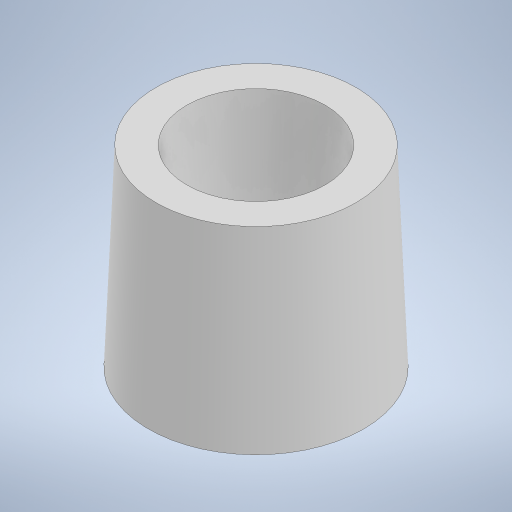
# Autodesk Inventor part: Washing Machine Base and Lid
Saved by Autodesk Inventor 2023 (Build 270158000, 158)
## iProperties
Created: 2023-08-28
Part Number: Washing Machine Base and Lid
Material: Generic
Document SubType Name: Modeling
Designer: tommy
Mass: 3317.36 g
Surface Area: 1872.07 cm^2
Volume: 3317.36 cm^3
Density: 1 g/cm^3
Appearance: Default
Author: tommy
Autodesk Inventor part; units mm, degrees
ref_plane "YZ Plane" through (0, 0, 0) normal (1, 0, 0) x (0, 1, 0)
ref_plane "XZ Plane" through (0, 0, 0) normal (0, 1, 0) x (-1, 0, 0)
ref_plane "XY Plane" through (0, 0, 0) normal (0, 0, 1) x (1, 0, 0)
sketch "Sketch1" plane through (0, 0, 0) normal (0, 0, 1) x (1, 0, 0)
  line L0 (0, 0) -> (0, 236.3219) construction
  line L1 (0, 0) -> (57.15, 0) construction
  line L2 (57.15, 0) -> (57.15, 158.75)
  line L3 (57.15, 158.75) -> (82.55, 158.75)
  line L4 (82.55, 158.75) -> (82.55, 0)
  line L5 (82.55, 0) -> (57.15, 0)
  line L6 (160.21, 0) -> (83.4701, 0)
  line L7 (0, 0) -> (0, 171.9026)
  line L8 (57.15, 158.75) -> (42.3187, 0)
  line L9 (106.8981, 0) -> (42.3187, 0)
  line L10 (57.15, 0) -> (88.9, 0)
  line L11 (88.9, 0) -> (82.55, 158.75)
  point P0 (83.4701, 0)
  point P1 (88.9, 0)
  point P2 (82.55, 0)
  dimension "d0" = 57.15
  dimension "d1" = 158.75
  dimension "d2" = 25.4
  dimension "d4" = 31.75
  constraints: 24 end point, 7 point on line, 4 perpendicular, 2 collinear, 1 horizontal, 1 vertical
  measures "d0" distance of L0.start L1.end
  measures "d1" distance of L1.end L2.end
  measures "d2" distance of L2.end L3.end
  measures "d4" distance of L1.end L10.end
revolve "Revolution1" add sketch "Sketch1" angle 360 about axis through (0, 0, 0) along (0, 1, 0)
body "Solid1"
